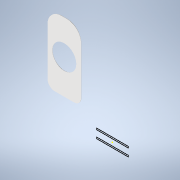
# Autodesk Inventor part: Bodenplatte-Holz
Saved by Autodesk Inventor 2020.3 (Build 243373010, 373A)
## iProperties
Created: 2021-01-31
Part Number: Bodenplatte-Holz
Material: Generisch
Document SubType Name: Modeling
Designer: Stefan
Density: 1 g/cm^3
Appearance: Vorgabe
Author: Stefan
Autodesk Inventor part; units mm, degrees
ref_plane "YZ Plane" through (0, 0, 0) normal (1, 0, 0) x (0, 1, 0)
ref_plane "XZ Plane" through (0, 0, 0) normal (0, 1, 0) x (-1, 0, 0)
ref_plane "XY Plane" through (0, 0, 0) normal (0, 0, 1) x (1, 0, 0)
sketch "Skizze2" plane through (0, 0, 0) normal (0, 0, 1) x (1, 0, 0)
  line L0 (-561.4045, 230.6141) -> (-561.4045, 1580.6141)
  line L1 (-161.4045, 1980.6141) -> (-11.4045, 1980.6141)
  line L2 (388.5955, 1580.6141) -> (388.5955, 230.6141)
  line L3 (188.5955, 30.6141) -> (-361.4045, 30.6141)
  arc A0 (-161.4045, 1980.6141) -> (-561.4045, 1580.6141) centre (-161.4045, 1580.6141) ccw
  arc A1 (388.5955, 1580.6141) -> (-11.4045, 1980.6141) centre (-11.4045, 1580.6141) ccw
  arc A2 (-561.4045, 230.6141) -> (-361.4045, 30.6141) centre (-361.4045, 230.6141) ccw
  arc A3 (188.5955, 30.6141) -> (388.5955, 230.6141) centre (188.5955, 230.6141) ccw
  circle A4 centre (-86.4045, 1005.6141) radius 340
  point P0 (388.5955, 1980.6141)
  point P1 (-561.4045, 1980.6141)
  point P2 (388.5955, 30.6141)
  dimension "d0" = 950
  dimension "d1" = 1950
  dimension "d2" = 400
  dimension "d3" = 200
  dimension "d4" = 680
  dimension "d17" = 475
  dimension "d18" = 975
  constraints: 8 end point, 8 point on circle, 8 tangent, 6 point on line, 5 centre point, 2 equal radius, 2 parallel, 1 coincident, 1 perpendicular, 1 vertical
  measures "d0" distance of point (-561.404, 1980.614) point (388.596, 1980.614)
  measures "d1" distance of point (388.596, 1980.614) point (388.596, 30.614)
  measures "d2" radius of A0
  measures "d3" radius of A2
  measures "d4" diameter of A4
  measures "d17" distance from line of L0 A4.centre
  measures "d18" distance from line of L1 A4.centre
extrude "Extrusion1" add sketch "Skizze2" along normal blind 10
sketch "Skizze3" plane through (0, 0, 10) normal (0, 0, 1) x (1, 0, 0)
  line L0 (43.5955, 1455.6141) -> (43.5955, 555.6141)
  line L1 (43.5955, 555.6141) -> (3.5955, 555.6141)
  line L2 (3.5955, 555.6141) -> (3.5955, 1455.6141)
  line L3 (3.5955, 1455.6141) -> (43.5955, 1455.6141)
  line L4 (-216.4045, 555.6141) -> (-216.4045, 1455.6141)
  line L5 (-216.4045, 1455.6141) -> (-176.4045, 1455.6141)
  line L6 (-176.4045, 1455.6141) -> (-176.4045, 555.6141)
  line L7 (-176.4045, 555.6141) -> (-216.4045, 555.6141)
  circle A0 centre (-86.4045, 1005.6141) radius 340 projected
  point P0 (0, 0)
  dimension "d9" = 900
  dimension "d10" = 40
  dimension "d13" = 900
  dimension "d14" = 40
  dimension "d20" = 260
  dimension "d21" = 0
  dimension "d23" = 130
  dimension "d24" = 450
  constraints: 16 end point, 4 parallel, 2 perpendicular, 2 vertical
  measures "d9" distance of L1.end L2.end
  measures "d10" distance of L0.end L1.end
  measures "d13" distance of L5.end L6.end
  measures "d14" distance of L4.end L5.end
  measures "d20" distance between parallel lines of L4 L0
  measures "d21" distance between parallel lines of L1 L7
  measures "d23" distance from line of A0.centre L4
  measures "d24" distance from line of A0.centre L1
